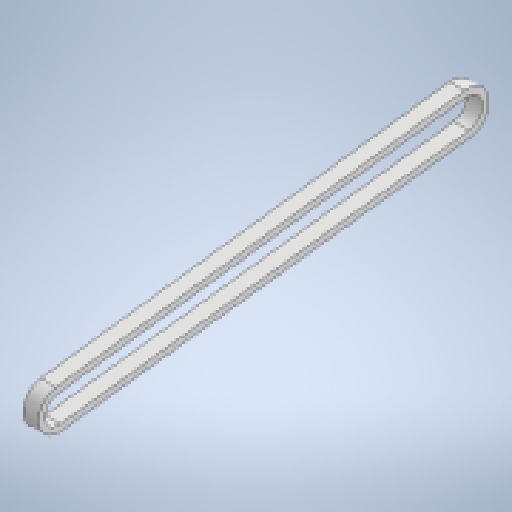
# Autodesk Inventor part: 112tooth belt
Saved by Autodesk Inventor 2023 (Build 270158000, 158)
## iProperties
Created: 2022-09-06
Part Number: 112tooth belt
Material: Generic
Document SubType Name: Modeling
Designer: deli
Density: 1 g/cm^3
Appearance: Default
Author: deli
Autodesk Inventor part; units mm, degrees
ref_plane "YZ Plane" through (0, 0, 0) normal (1, 0, 0) x (0, 1, 0)
ref_plane "XZ Plane" through (0, 0, 0) normal (0, 1, 0) x (-1, 0, 0)
ref_plane "XY Plane" through (0, 0, 0) normal (0, 0, 1) x (1, 0, 0)
sketch "Sketch1" plane through (0, 0, 0) normal (1, 0, 0) x (0, 1, 0)
  circle A0 centre (20.621, 120.258) radius 2 construction
  circle A1 centre (47.871, -119.5312) radius 7 construction
  arc A2 (35.2153, -120.9272) -> (60.5171, -118.0519) centre (47.871, -119.5312) ccw
  arc A3 (32.4767, 121.6449) -> (8.7563, 118.9493) centre (20.621, 120.258) ccw
  line L0 (60.5171, -118.0519) -> (32.4767, 121.6449)
  line L1 (8.7563, 118.9493) -> (35.2153, -120.9272)
  line L2 (28.7025, 121.2034) -> (56.7429, -118.4934)
  arc A4 (38.9924, -120.5106) -> (56.7429, -118.4934) centre (47.871, -119.5312) ccw
  line L3 (38.9924, -120.5106) -> (12.5334, 119.3659)
  arc A5 (28.7025, 121.2034) -> (12.5334, 119.3659) centre (20.621, 120.258) ccw
  point P0 (0, 0)
  dimension "d0" = 25.4648
  dimension "d1" = 23.8732
  dimension "d2" = 3.8
  constraints: 8 end point, 8 point on circle, 4 centre point, 4 tangent, 2 coincident, 3 other
  measures "d0" diameter of A2
  measures "d1" diameter of A3
  measures "d2" distance between parallel lines of L0 L2
extrude "Extrusion1" add sketch "Sketch1" along normal blind 9
body "Solid1"
